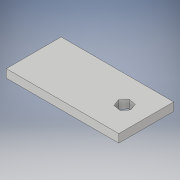
# Autodesk Inventor part: back
Saved by Autodesk Inventor 2019 (Build 230136000, 136)
## iProperties
Created: 2023-04-15
Part Number: back
Material: Generic
Document SubType Name: Modeling
Designer: Analuam
Density: 1 g/cm^3
Appearance: Default
Author: Analuam
Autodesk Inventor part; units mm, degrees
ref_plane "YZ Plane" through (0, 0, 0) normal (1, 0, 0) x (0, 1, 0)
ref_plane "XZ Plane" through (0, 0, 0) normal (0, 1, 0) x (-1, 0, 0)
ref_plane "XY Plane" through (0, 0, 0) normal (0, 0, 1) x (1, 0, 0)
sketch "Sketch1" plane through (0, 0, 0) normal (0, 1, 0) x (-1, 0, 0)
  line L0 (19.0624, 34.842) -> (-21.9376, 34.842)
  line L1 (-21.9376, 34.842) -> (-21.9376, 14.842)
  line L2 (-21.9376, 14.842) -> (19.0624, 14.842)
  line L3 (19.0624, 14.842) -> (19.0624, 34.842)
  circle A0 centre (-13.9376, 24.7364) radius 1.5
  line L4 (-11.2365, 24.2625) -> (-12.9974, 22.1601)
  line L5 (-12.9974, 22.1601) -> (-15.6986, 22.634)
  line L6 (-15.6986, 22.634) -> (-16.6388, 25.2103)
  line L7 (-16.6388, 25.2103) -> (-14.8778, 27.3126)
  line L8 (-14.8778, 27.3126) -> (-12.1767, 26.8387)
  line L9 (-12.1767, 26.8387) -> (-11.2365, 24.2625)
  point P0 (0, 0)
  dimension "d0" = 41
  dimension "d1" = 20
  dimension "d2" = 3
  dimension "d3" = 8
  dimension "d6" = 4.75
  constraints: 20 end point, 2 parallel, 1 centre point, 1 coincident, 1 horizontal, 1 perpendicular, 13 other
  measures "d0" distance of L2.end L1.end
  measures "d1" distance of L1.end L0.end
  measures "d2" diameter of A0
  measures "d3" distance from line of L1 A0.centre
  measures "d6" distance between parallel lines of L7 L4
extrude "Extrusion2" add sketch "Sketch1" along normal blind 3 contours L3 L2 L1 L0
body "Solid2"
